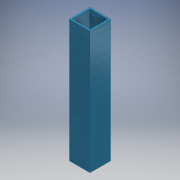
# Autodesk Inventor part: bogie_bar_sample_300
Saved by Autodesk Inventor 2018 (Build 220112000, 112)
## iProperties
Created: 2017-10-24
Part Number: bogie_bar_sample_300
Material: アルミニウム 6061
Document SubType Name: Modeling
Designer: 翔
Density: 2.7 g/cm^3
Appearance: スカイ ブルー 濃い
Author: 翔
Autodesk Inventor part; units mm, degrees
ref_plane "YZ Plane" through (0, 0, 0) normal (1, 0, 0) x (0, 1, 0)
ref_plane "XZ Plane" through (0, 0, 0) normal (0, 1, 0) x (-1, 0, 0)
ref_plane "XY Plane" through (0, 0, 0) normal (0, 0, 1) x (1, 0, 0)
sketch "スケッチ1" plane through (0, 0, 0) normal (0, 0, 1) x (1, 0, 0)
  line L0 (-25, -25) -> (25, -25)
  line L1 (25, -25) -> (25, 25)
  line L2 (25, 25) -> (-25, 25)
  line L3 (-25, 25) -> (-25, -25)
  line L4 (-25, -25) -> (25, 25) construction
  line L5 (25, -25) -> (-25, 25) construction
  line L6 (-22, 22) -> (22, 22)
  line L7 (22, 22) -> (22, -22)
  line L8 (22, -22) -> (-22, -22)
  line L9 (-22, -22) -> (-22, 22)
  point P0 (0, 0)
  dimension "d0" = 50
  dimension "d1" = 50
  dimension "d2" = 3
  constraints: 20 end point, 4 parallel, 2 midpoint, 2 perpendicular, 1 horizontal, 3 other
  measures "d0" distance of L1.end L2.end
  measures "d1" distance of L0.end L1.end
  measures "d2" distance between parallel lines of L6 L2
extrude "押し出し1" add sketch "スケッチ1" along normal blind 300
sketch "スケッチ2" plane through (-25, 25, 0) normal (0, 1, 0) x (1, 0, 0)
  line L0 (0, 0) -> (0, -300) projected
  line L1 (50, 0) -> (0, 0) projected
  line L2 (40, -40) -> (10, -40)
  line L3 (10, -40) -> (10, -10)
  line L4 (10, -10) -> (40, -10)
  line L5 (40, -10) -> (40, -40)
  line L6 (40, -40) -> (10, -10) construction
  line L7 (10, -40) -> (40, -10) construction
  circle A0 centre (10, -10) radius 2.5
  circle A1 centre (40, -10) radius 2.5
  circle A2 centre (10, -40) radius 2.5
  circle A3 centre (40, -40) radius 2.5
  line L8 (40, -290) -> (10, -290)
  line L9 (10, -290) -> (10, -260)
  line L10 (10, -260) -> (40, -260)
  line L11 (40, -260) -> (40, -290)
  line L12 (40, -290) -> (10, -260) construction
  line L13 (10, -290) -> (40, -260) construction
  line L14 (50, -300) -> (0, -300) projected
  circle A4 centre (10, -290) radius 2.5
  circle A5 centre (10, -260) radius 2.5
  circle A6 centre (40, -290) radius 2.5
  circle A7 centre (40, -260) radius 2.5
  point P0 (25, 0)
  point P1 (25, -25)
  point P2 (25, -275)
  dimension "d8" = 30
  dimension "d9" = 30
  dimension "d10" = 25
  dimension "d12" = 10
  dimension "d13" = 5
  dimension "d16" = 30
  dimension "d19" = 30
  dimension "d22" = 30
  dimension "d23" = 30
  dimension "d24" = 10
  dimension "d25" = 10
  dimension "d26" = 5
  dimension "d29" = 30
  dimension "d32" = 30
  constraints: 24 end point, 8 centre point, 4 horizontal, 4 midpoint, 4 parallel, 2 coincident, 2 perpendicular, 2 vertical, 12 other
  measures "d8" distance of L3.end L4.end
  measures "d9" distance of L2.end L3.end
  measures "d10" distance from line of point (25, -25) L0
  measures "d12" distance between parallel lines of L4 L1
  measures "d13" diameter of A0
  measures "d16" distance of A0.centre A1.centre
  measures "d19" distance of A0.centre A2.centre
  measures "d22" distance of L9.end L10.end
  measures "d23" distance of L8.end L9.end
  measures "d24" distance between parallel lines of L9 L0
  measures "d25" distance between parallel lines of L8 L14
  measures "d26" diameter of A4
  measures "d29" distance of A4.centre A5.centre
  measures "d32" distance of A4.centre A6.centre
extrude "押し出し2" cut sketch "スケッチ2" against normal through all contours A2 L3 L2 | L2 L3 A2 | A3 L5 L2 | L2 L5 A3 | A0 L4 L3 | L3 L4 A0 | A1 L4 L5 | L5 L4 A1 | A4 L9 L8 | L8 L9 A4 | A6 L11 L8 | L8 L11 A6 | A5 L10 L9 | L9 L10 A5 | A7 L10 L11 | L11 L10 A7
